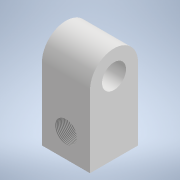
# Autodesk Inventor part: klocek
Saved by Autodesk Inventor 2021 (Build 250183000, 183)
## iProperties
Created: 2021-10-08
Part Number: klocek
Material: Generic
Document SubType Name: Modeling
Designer: nikod
Density: 1 g/cm^3
Appearance: Default
Author: nikod
Autodesk Inventor part; units mm, degrees
ref_plane "YZ Plane" through (0, 0, 0) normal (1, 0, 0) x (0, 1, 0)
ref_plane "XZ Plane" through (0, 0, 0) normal (0, 1, 0) x (-1, 0, 0)
ref_plane "XY Plane" through (0, 0, 0) normal (0, 0, 1) x (1, 0, 0)
sketch "Sketch1" plane through (0, 0, 0) normal (0, 0, 1) x (1, 0, 0)
  line L0 (3.5859, 14.3435) -> (203.5859, 14.3435)
  line L1 (203.5859, 14.3435) -> (203.5859, -185.6565)
  line L2 (203.5859, -185.6565) -> (3.5859, -185.6565)
  line L3 (3.5859, -185.6565) -> (3.5859, 14.3435)
  point P0 (0, 0)
  dimension "d0" = 200
  dimension "d1" = 200
  constraints: 8 end point, 2 parallel, 1 horizontal, 1 perpendicular
  measures "d0" distance of L1.end L2.end
  measures "d1" distance of L0.end L1.end
extrude "Extrusion1" add sketch "Sketch1" along normal blind 200
sketch "Sketch2" plane through (0, 0, 200) normal (0, 0, 1) x (1, 0, 0)
  line L0 (203.5859, 14.3435) -> (3.5859, 14.3435) projected
  line L1 (3.5859, -185.6565) -> (203.5859, -185.6565) projected
  circle A0 centre (103.5859, -85.6565) radius 45
  point P0 (0, 0)
  dimension "d4" = 90
  constraints: 1 centre point
  measures "d4" diameter of A0
extrude "Extrusion2" cut sketch "Sketch2" against normal blind 200
thread "Thread1" size "M90x6" class "6H" standard "ANSI Metric M Profile" full length
sketch "Sketch3" plane through (3.5859, 14.3435, 0) normal (0, 1, 0) x (1, 0, 0)
  line L0 (0, -200) -> (200, -200) projected
  line L1 (200, 0) -> (200, -200) projected
  line L2 (0, -200) -> (200, -200)
  line L3 (200, -200) -> (200, 0)
  line L4 (200, 0) -> (0, 0)
  line L5 (0, 0) -> (0, -200)
  point P0 (-3.5859, 0)
  constraints: 8 end point, 2 parallel, 1 horizontal, 1 perpendicular
extrude "Extrusion3" add sketch "Sketch3" along normal blind 200
fillet "Fillet1" radius 100 2 edges at (103.5859, 214.3435, 0) (103.5859, 214.3435, 200)
sketch "Sketch4" plane through (3.5859, -185.6565, 0) normal (-1, 0, 0) x (0, 0, 1)
  arc A0 (200, 300) -> (0, 300) centre (100, 300) ccw projected
  circle A1 centre (100, 300) radius 25
  point P0 (0, 185.6565)
  dimension "d12" = 50
  constraints: 1 centre point, 1 coincident
  measures "d12" diameter of A1
hole "Hole1" at (3.5859, 114.3435, 100) direction (1, 0, 0) diameter 100 end through all
body "Solid1"
